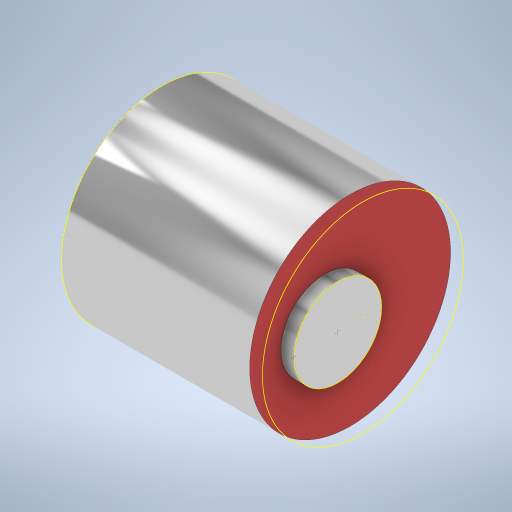
# Autodesk Inventor part: Przekładnia rolka
Saved by Autodesk Inventor 2023 (Build 270158000, 158)
## iProperties
Created: 2023-04-01
Part Number: Przekładnia rolka
Material: Stal
Document SubType Name: Modeling
Designer: Wiktor
Density: 7.85 g/cm^3
Appearance: Chrom — polerowany
Author: Wiktor
Autodesk Inventor part; units mm, degrees
ref_plane "YZ Plane" through (0, 0, 0) normal (1, 0, 0) x (0, 1, 0)
ref_plane "XZ Plane" through (0, 0, 0) normal (0, 1, 0) x (-1, 0, 0)
ref_plane "XY Plane" through (0, 0, 0) normal (0, 0, 1) x (1, 0, 0)
sketch "Szkic1" plane through (0, 0, 0) normal (1, 0, 0) x (0, 1, 0)
  circle A0 centre (0, 0) radius 8
  dimension "d0" = 16
  constraints: 1 centre point, 1 coincident
  measures "d0" diameter of A0
extrude "Wyciągnięcie proste1" add sketch "Szkic1" along normal mid plane 15
sketch "Szkic2" plane through (7.5, 0, 0) normal (1, 0, 0) x (0, 0, -1)
  circle A0 centre (-2, 0) radius 3.5
  point P0 (0, 0)
  dimension "d3" = 7
  dimension "d4" = 2
  constraints: 1 centre point, 1 horizontal alignment
  measures "d3" diameter of A0
  measures "d4" distance of point (0, 0) A0.centre
extrude "Wyciągnięcie proste2" add sketch "Szkic2" along normal blind 1
mirror "Odbij1" about plane through (0, 0, 0) normal (1, 0, 0) of "Wyciągnięcie proste2", "Wyciągnięcie proste1"
sketch "Szkic3" plane through (7.5, 0, 0) normal (1, 0, 0) x (0, 0, -1)
  point P0 (0, 0)
sketch "Szkic4" plane through (8.5, 0, 2) normal (1, 0, 0) x (0, 0, -1)
  circle A0 centre (2, 0) radius 8 projected
  circle A1 centre (0, 0) radius 3.5 projected
  point P0 (-6, 0)
  point P1 (-3.5, 0)
  constraints: 2 horizontal alignment, 2 other
sketch "Szkic8" plane through (-7.5, 0, 0) normal (-1, 0, 0) x (0, 0, 1)
  circle A0 centre (0, 0) radius 8 projected
  line L0 (8, 0) -> (5.5, 0)
  circle A1 centre (2, 0) radius 3.5 projected
  constraints: 2 end point, 2 horizontal alignment, 1 horizontal, 2 other
